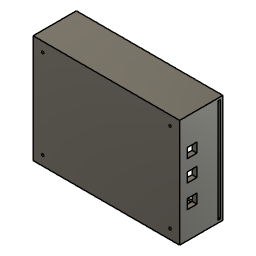
Shades+PCB+Holder+#2 (Autodesk Fusion 360 design; units mm, degrees)
Autodesk Fusion 360 part; units mm, degrees
note: some values were not read from the file. Set by a fixed rule: which sketch regions a step uses.
sketch "Sketch1" plane through (0, 0, 0) normal (0, 0, 1) x (1, 0, 0)
  line L0 (0, 0) -> (-152.5, 0)
  line L1 (-152.5, 0) -> (-152.5, 112.5)
  line L2 (-152.5, 112.5) -> (0, 112.5)
  line L3 (0, 112.5) -> (0, 0)
  line L4 (-152.5, 112.5) -> (-147.5, 112.5)
  line L5 (0, 0) -> (0, 5)
  line L6 (-147.5, 107.5) -> (-5, 107.5)
  line L7 (-5, 107.5) -> (-5, 5)
  line L8 (-5, 5) -> (-147.5, 5)
  line L9 (-147.5, 5) -> (-147.5, 107.5)
  dimension "d1" = 152.5
  dimension "d2" = 112.5
  dimension "d3" = 5
  dimension "d4" = 5
  dimension "d5" = 5
  dimension "d6" = 5
  constraint horizontal L0
  constraint vertical L1
  constraint horizontal L2
  constraint vertical L3
  constraint coincident L0.start L3.end
  constraint perpendicular L1 L4
  constraint perpendicular L0 L5
  constraint horizontal L6
  constraint vertical L7
  constraint horizontal L8
  constraint vertical L9
  measures "d1" distance of L0.start L0.end
  measures "d2" distance of L0.start L2.end
  measures "d3" distance of L1.end L4.end
  measures "d4" distance of L4.end L6.start
  measures "d5" distance of L0.start L5.end
  measures "d6" distance of L5.end L7.end
extrude "Extrude1" add sketch "Sketch1" along normal blind 5 contours L0 L1 L2 L3 L4 L5 | L6 L7 L8 L9
sketch "Sketch2" plane through (0, 0, 0) normal (0, 0, -1) x (-1, 0, 0)
  line L0 (0, 0) -> (152.5, 0)
  line L1 (152.5, 0) -> (152.5, 112.5)
  line L2 (152.5, 112.5) -> (0, 112.5)
  line L3 (0, 112.5) -> (0, 0)
  line L4 (152.5, 112.5) -> (147.5, 112.5)
  line L5 (147.5, 112.5) -> (147.5, 107.5)
  line L6 (0, 0) -> (0, 5)
  line L7 (0, 5) -> (5, 5)
  line L8 (147.5, 107.5) -> (5, 107.5)
  line L9 (5, 107.5) -> (5, 5)
  line L10 (5, 5) -> (147.5, 5)
  line L11 (147.5, 5) -> (147.5, 107.5)
  dimension "d9" = 5
  dimension "d10" = 5
  dimension "d11" = 5
  constraint coincident L1.end L2.start
  constraint perpendicular L1 L4
  constraint perpendicular L4 L5
  constraint coincident L0.start L3.end
  constraint perpendicular L0 L6
  constraint perpendicular L6 L7
  constraint horizontal L8
  constraint vertical L9
  constraint horizontal L10
  constraint vertical L11
  measures "d9" distance of L1.end L4.end
  measures "d10" distance of L4.end L5.end
  measures "d11" distance of L0.start L6.end
extrude "Extrude2" add sketch "Sketch2" along normal blind 25 contours L0 L1 L2 L3 L4 L5 L6 L7 L10 L11 | L2 L3 L5 L7 L8 L9
sketch "Sketch3" plane through (0, 0, 0) normal (1, 0, 0) x (0, 0, -1)
  line L0 (25, 112.5) -> (-5, 112.5)
  line L1 (-5, 112.5) -> (-5, 0)
  line L2 (-5, 0) -> (25, 0)
  line L3 (25, 0) -> (25, 112.5)
  line L4 (-5, 0) -> (-5, 20)
  line L5 (-5, 20) -> (-5, 45)
  line L6 (-5, 45) -> (-5, 70)
  line L7 (-5, 70) -> (10, 70)
  line L8 (-5, 45) -> (10, 45)
  line L9 (-5, 20) -> (10, 20)
  line L10 (10, 70) -> (10, 75)
  line L11 (10, 70) -> (10, 65)
  line L12 (10, 45) -> (10, 50)
  line L13 (10, 45) -> (10, 40)
  line L14 (10, 20) -> (10, 25)
  line L15 (10, 20) -> (10, 15)
  line L16 (10, 75) -> (5, 75)
  line L17 (10, 65) -> (15, 65)
  line L18 (10, 50) -> (5, 50)
  line L19 (10, 40) -> (15, 40)
  line L20 (10, 25) -> (5, 25)
  line L21 (10, 15) -> (15, 15)
  line L22 (5, 75) -> (15, 75)
  line L23 (15, 75) -> (15, 65)
  line L24 (15, 65) -> (5, 65)
  line L25 (5, 65) -> (5, 75)
  line L26 (5, 50) -> (15, 50)
  line L27 (15, 50) -> (15, 40)
  line L28 (15, 40) -> (5, 40)
  line L29 (5, 40) -> (5, 50)
  line L30 (5, 25) -> (15, 25)
  line L31 (15, 25) -> (15, 15)
  line L32 (15, 15) -> (5, 15)
  line L33 (5, 15) -> (5, 25)
  dimension "d14" = 25
  dimension "d15" = 5
  dimension "d16" = 5
  dimension "d17" = 5
  dimension "d18" = 5
  dimension "d19" = 5
  dimension "d20" = 5
  dimension "d21" = 5
  dimension "d22" = 5
  dimension "d23" = 5
  dimension "d24" = 5
  constraint coincident L1.end L2.start
  constraint coincident L1 L4.end
  constraint perpendicular L2 L4
  constraint perpendicular L2 L5
  constraint coincident L1 L6.end
  constraint parallel L1 L6
  constraint perpendicular L6 L7
  constraint perpendicular L5 L8
  constraint perpendicular L6 L9
  constraint perpendicular L7 L10
  constraint perpendicular L7 L11
  constraint perpendicular L8 L12
  constraint perpendicular L8 L13
  constraint perpendicular L9 L14
  constraint perpendicular L9 L15
  constraint perpendicular L10 L16
  constraint perpendicular L11 L17
  constraint perpendicular L12 L18
  constraint perpendicular L13 L19
  constraint perpendicular L14 L20
  constraint perpendicular L15 L21
  constraint horizontal L22
  constraint vertical L23
  constraint horizontal L24
  constraint vertical L25
  constraint horizontal L26
  constraint vertical L27
  constraint horizontal L28
  constraint vertical L29
  constraint horizontal L30
  constraint vertical L31
  constraint horizontal L32
  constraint vertical L33
  measures "d14" distance of L4.end L5.end
  measures "d15" distance of L7.end L10.end
  measures "d16" distance of L7.end L11.end
  measures "d17" distance of L9.end L14.end
  measures "d18" distance of L9.end L15.end
  measures "d19" distance of L10.end L16.end
  measures "d20" distance of L11.end L17.end
  measures "d21" distance of L12.end L18.end
  measures "d22" distance of L13.end L19.end
  measures "d23" distance of L14.end L20.end
  measures "d24" distance of L15.end L21.end
extrude "Extrude3" cut sketch "Sketch3" against normal blind 10 contours L7 L10 L16 L22 L25 | L7 L11 L24 L25 | L10 L11 L17 L22 L23 L24 | L8 L12 L18 L26 L29 | L8 L13 L28 L29 | L12 L13 L19 L26 L27 L28 | L9 L14 L20 L30 L33 | L9 L15 L32 L33 | L14 L15 L21 L30 L31 L32
sketch "Sketch4" plane through (0, 0, 0) normal (0, 0, -1) x (-1, 0, 0)
  line L0 (147.5, 107.5) -> (5, 107.5)
  line L1 (5, 107.5) -> (5, 5)
  line L2 (5, 5) -> (147.5, 5)
  line L3 (147.5, 5) -> (147.5, 107.5)
  line L4 (5, 107.5) -> (5, 102.5)
  line L5 (5, 5) -> (5, 10)
  line L6 (10, 10) -> (142.5, 10)
  line L7 (10, 102.5) -> (142.5, 102.5)
  line L8 (142.5, 102.5) -> (142.5, 10)
  line L9 (10, 102.5) -> (10, 10)
  circle A0 centre (10, 102.5) radius 1.25
  circle A1 centre (10, 10) radius 1.25
  circle A2 centre (142.5, 10) radius 1.25
  circle A3 centre (142.5, 102.5) radius 1.25
  dimension "d27" = 5
  dimension "d28" = 132.5
  dimension "d29" = 132.5
  dimension "d30" = 2.5
  dimension "d31" = 2.5
  dimension "d32" = 2.5
  dimension "d33" = 2.5
  constraint coincident L0.end L1.start
  constraint perpendicular L0 L4
  constraint coincident L1.end L2.start
  constraint coincident L1 L5.end
  constraint perpendicular L2 L5
  constraint perpendicular L1 L6
  constraint parallel L0 L7
  constraint perpendicular L6 L8
  constraint coincident L7.start L9.start
  constraint coincident L6.start L9.end
  constraint coincident L6.end L8.end
  constraint coincident L7.end L8.start
  measures "d27" distance of L0.end L4.end
  measures "d28" distance of L6.start L6.end
  measures "d29" distance of L7.start L7.end
  measures "d30" diameter of A0
  measures "d31" diameter of A1
  measures "d32" diameter of A2
  measures "d33" diameter of A3
extrude "Extrude4" cut sketch "Sketch4" against normal blind 20 contours L6 L9 A1 | L6 L9 A1 | L6 L8 A2 | L6 L8 A2 | L7 L9 A0 | L7 L9 A0 | L7 L8 A3 | L7 L8 A3
extrude "Extrude5" add 1 faces at (-54.5498, 41.1167, 5) along direction (0, 0, 1) blind 10
sketch "Sketch5" plane through (0, 0, 0) normal (1, 0, 0) x (0, 0, -1)
  line L0 (15, 25) -> (15, 15)
  line L1 (15, 15) -> (5, 15)
  line L2 (5, 15) -> (5, 25)
  line L3 (5, 25) -> (15, 25)
  line L4 (15, 50) -> (15, 40)
  line L5 (15, 40) -> (5, 40)
  line L6 (5, 40) -> (5, 50)
  line L7 (5, 50) -> (15, 50)
  line L8 (15, 75) -> (15, 65)
  line L9 (15, 65) -> (5, 65)
  line L10 (5, 65) -> (5, 75)
  line L11 (5, 75) -> (15, 75)
  line L12 (25, 112.5) -> (-15, 112.5)
  line L13 (-15, 112.5) -> (-15, 0)
  line L14 (-15, 0) -> (25, 0)
  line L15 (25, 0) -> (25, 112.5)
  line L16 (25, 112.5) -> (22.5, 112.5)
  line L17 (22.5, 112.5) -> (22.5, 110)
  line L18 (25, 0) -> (22.5, 0)
  line L19 (22.5, 0) -> (22.5, 2.5)
  line L20 (22.5, 110) -> (20, 110)
  line L21 (22.5, 2.5) -> (20, 2.5)
  line L22 (22.5, 110) -> (20, 110)
  line L23 (20, 110) -> (20, 2.5)
  line L24 (20, 2.5) -> (22.5, 2.5)
  line L25 (22.5, 2.5) -> (22.5, 110)
  dimension "d38" = 2.5
  dimension "d39" = 2.5
  dimension "d40" = 2.5
  constraint coincident L12.start L15.end
  constraint perpendicular L15 L16
  constraint perpendicular L12 L17
  constraint coincident L14.end L15.start
  constraint perpendicular L15 L18
  constraint perpendicular L14 L19
  constraint perpendicular L17 L20
  constraint perpendicular L15 L21
  constraint horizontal L22
  constraint vertical L23
  constraint horizontal L24
  constraint vertical L25
  measures "d38" distance of L12.start L16.end
  measures "d39" distance of L14.end L18.end
  measures "d40" distance of L18.end L19.end
extrude "Extrude6" cut sketch "Sketch5" against normal blind 150.5 contours L20 L21 L22 L23 L24 L25
extrude "Extrude7" cut 1 faces at (-147.5, 39.1667, -23.3333) along direction (-1, 0, 0) blind 1
extrude "Extrude8" cut 1 faces at (-148.5, 39.1667, -23.3333) along direction (-1, 0, 0) blind 1
extrude "Extrude9" cut 1 faces at (-150.5, 74.1667, -20.8333) along direction (-1, 0, 0) blind 1
extrude "Extrude10" cut 1 faces at (-101.3333, 107.5, -23.3333) along direction (0, 1, 0) blind 3
extrude "Extrude11" cut 1 faces at (-53.1667, 5, -24.1667) along direction (0, -1, 0) blind 3
extrude "Extrude12" add 1 faces at (-54.5498, 41.1167, 15) along direction (0, 0, 1) blind 5
extrude "Extrude13" cut 1 faces at (-54.5555, 41.0963, 0) along direction (0, 0, 1) blind 15
sketch "Sketch6" plane through (0, 0, 0) normal (1, 0, 0) x (0, 0, -1)
  line L0 (20, 110) -> (22.5, 110)
  line L1 (22.5, 110) -> (22.5, 2.5)
  line L2 (22.5, 2.5) -> (20, 2.5)
  line L3 (20, 2.5) -> (20, 110)
  line L4 (15, 25) -> (15, 15)
  line L5 (15, 15) -> (5, 15)
  line L6 (5, 15) -> (5, 25)
  line L7 (5, 25) -> (15, 25)
  line L8 (15, 50) -> (15, 40)
  line L9 (15, 40) -> (5, 40)
  line L10 (5, 40) -> (5, 50)
  line L11 (5, 50) -> (15, 50)
  line L12 (15, 75) -> (15, 65)
  line L13 (15, 65) -> (5, 65)
  line L14 (5, 65) -> (5, 75)
  line L15 (5, 75) -> (15, 75)
  line L16 (25, 112.5) -> (-20, 112.5)
  line L17 (-20, 112.5) -> (-20, 0)
  line L18 (-20, 0) -> (25, 0)
  line L19 (25, 0) -> (25, 112.5)
sketch "Sketch7" plane through (0, 0, 0) normal (1, 0, 0) x (0, 0, -1)
sketch "Sketch8" plane through (0, 0, 0) normal (1, 0, 0) x (0, 0, -1)
  line L0 (-14, 84) -> (-4, 84)
  line L1 (-4, 84) -> (-4, 74)
  line L2 (-4, 74) -> (-14, 74)
  line L3 (-14, 74) -> (-14, 84)
  line L4 (-14, 62) -> (-4, 62)
  line L5 (-4, 62) -> (-4, 52)
  line L6 (-4, 52) -> (-14, 52)
  line L7 (-14, 52) -> (-14, 62)
  line L8 (-14, 38) -> (-4, 38)
  line L9 (-4, 38) -> (-4, 28)
  line L10 (-4, 28) -> (-14, 28)
  line L11 (-14, 28) -> (-14, 38)
  constraint horizontal L0
  constraint vertical L1
  constraint horizontal L2
  constraint vertical L3
  constraint horizontal L4
  constraint vertical L5
  constraint horizontal L6
  constraint vertical L7
  constraint horizontal L8
  constraint vertical L9
  constraint horizontal L10
  constraint vertical L11
extrude "Extrude14" add sketch "Sketch6" against normal blind 5 contours L4 L5 L6 L7 | L8 L9 L10 L11 | L12 L13 L14 L15
extrude "Extrude15" cut sketch "Sketch8" against normal blind 5
sketch "Sketch9" plane through (-152.5, 0, 0) normal (-1, 0, 0) x (0, 0, 1)
  line L0 (-25, 0) -> (20, 0)
  line L1 (20, 0) -> (20, 112.5)
  line L2 (20, 112.5) -> (-25, 112.5)
  line L3 (-25, 112.5) -> (-25, 0)
  line L4 (12, 15) -> (-2, 15)
  line L5 (-2, 15) -> (-2, 40)
  line L6 (-2, 40) -> (12, 40)
  line L7 (12, 40) -> (12, 15)
  constraint horizontal L4
  constraint vertical L5
  constraint horizontal L6
  constraint vertical L7
extrude "Extrude16" cut sketch "Sketch9" against normal blind 5 contours L4 L5 L6 L7
sketch "Sketch10" plane through (0, 0, 0) normal (1, 0, 0) x (0, 0, -1)
  line L0 (-4, 84) -> (-4, 74)
  line L1 (-4, 74) -> (-14, 74)
  line L2 (-14, 74) -> (-14, 84)
  line L3 (-14, 84) -> (-4, 84)
  line L4 (-4, 62) -> (-4, 52)
  line L5 (-4, 52) -> (-14, 52)
  line L6 (-14, 52) -> (-14, 62)
  line L7 (-14, 62) -> (-4, 62)
  line L8 (-4, 38) -> (-4, 28)
  line L9 (-4, 28) -> (-14, 28)
  line L10 (-14, 28) -> (-14, 38)
  line L11 (-14, 38) -> (-4, 38)
  line L12 (20, 110) -> (22.5, 110)
  line L13 (22.5, 110) -> (22.5, 2.5)
  line L14 (22.5, 2.5) -> (20, 2.5)
  line L15 (20, 2.5) -> (20, 110)
  line L16 (25, 112.5) -> (-20, 112.5)
  line L17 (-20, 112.5) -> (-20, 0)
  line L18 (-20, 0) -> (25, 0)
  line L19 (25, 0) -> (25, 112.5)
  line L20 (-4, 84) -> (-2, 84)
  line L21 (-2, 84) -> (-2, 74)
  line L22 (-2, 74) -> (-4, 74)
  line L23 (-4, 74) -> (-4, 84)
  line L24 (-4, 62) -> (-2, 62)
  line L25 (-2, 62) -> (-2, 52)
  line L26 (-2, 52) -> (-4, 52)
  line L27 (-4, 52) -> (-4, 62)
  line L28 (-4, 38) -> (-2, 38)
  line L29 (-2, 38) -> (-2, 28)
  line L30 (-2, 28) -> (-4, 28)
  line L31 (-4, 28) -> (-4, 38)
  line L32 (-14, 28) -> (-12, 28)
  line L33 (-12, 28) -> (-12, 84)
  line L34 (-12, 84) -> (-14, 84)
  line L35 (-14, 84) -> (-14, 28)
  constraint horizontal L20
  constraint vertical L21
  constraint horizontal L22
  constraint vertical L23
  constraint coincident L0.start L3.end
  constraint horizontal L24
  constraint vertical L25
  constraint horizontal L26
  constraint vertical L27
  constraint coincident L4.start L7.end
  constraint horizontal L28
  constraint vertical L29
  constraint horizontal L30
  constraint vertical L31
  constraint coincident L8.start L11.end
  constraint horizontal L32
  constraint vertical L33
  constraint horizontal L34
  constraint vertical L35
  constraint coincident L3 L33.end
  constraint coincident L9.end L10.start
extrude "Extrude17" add sketch "Sketch10" against normal blind 5 contours L1 L2 L3 L33 L34 L35 | L5 L6 L7 L33 L35 | L9 L10 L11 L32 L33 L35
sketch "Sketch11" plane through (0, 0, 0) normal (1, 0, 0) x (0, 0, -1)
  line L0 (-4, 84) -> (-4, 74)
  line L1 (-4, 74) -> (-12, 74)
  line L2 (-12, 74) -> (-12, 84)
  line L3 (-12, 84) -> (-4, 84)
  line L4 (-4, 62) -> (-4, 52)
  line L5 (-4, 52) -> (-12, 52)
  line L6 (-12, 52) -> (-12, 62)
  line L7 (-12, 62) -> (-4, 62)
  line L8 (-4, 38) -> (-4, 28)
  line L9 (-4, 28) -> (-12, 28)
  line L10 (-12, 28) -> (-12, 38)
  line L11 (-12, 38) -> (-4, 38)
  line L12 (20, 110) -> (22.5, 110)
  line L13 (22.5, 110) -> (22.5, 2.5)
  line L14 (22.5, 2.5) -> (20, 2.5)
  line L15 (20, 2.5) -> (20, 110)
  line L16 (25, 112.5) -> (-20, 112.5)
  line L17 (-20, 112.5) -> (-20, 0)
  line L18 (-20, 0) -> (25, 0)
  line L19 (25, 0) -> (25, 112.5)
  line L20 (-4, 62) -> (-2, 62)
  line L21 (-2, 62) -> (-2, 52)
  line L22 (-2, 52) -> (-4, 52)
  line L23 (-4, 52) -> (-4, 62)
  line L24 (-4, 38) -> (-2, 38)
  line L25 (-2, 38) -> (-2, 28)
  line L26 (-2, 28) -> (-4, 28)
  line L27 (-4, 28) -> (-4, 38)
  line L28 (-4, 84) -> (-2, 84)
  line L29 (-2, 84) -> (-2, 74)
  line L30 (-2, 74) -> (-4, 74)
  line L31 (-4, 74) -> (-4, 84)
  constraint horizontal L20
  constraint vertical L21
  constraint horizontal L22
  constraint vertical L23
  constraint coincident L4.start L7.end
  constraint horizontal L24
  constraint vertical L25
  constraint horizontal L26
  constraint vertical L27
  constraint coincident L8.start L11.end
  constraint horizontal L28
  constraint vertical L29
  constraint horizontal L30
  constraint vertical L31
  constraint coincident L0.start L3.end
extrude "Extrude18" cut sketch "Sketch11" against normal blind 5 contours L0 L28 L29 L30 L31 | L4 L20 L21 L22 L23 | L8 L24 L25 L26 L27
